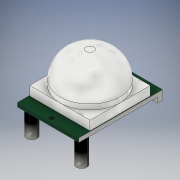
# Autodesk Inventor part: MotionSensor
Saved by Autodesk Inventor 2017.2 (Build 212223000, 223)
## iProperties
Created: 2017-02-21
Part Number: MotionSensor
Material: Generic
Document SubType Name: Modeling
Designer: prosp
Density: 1 g/cm^3
Appearance: Default
Author: prosp
Autodesk Inventor part; units mm, degrees
ref_plane "YZ Plane" through (0, 0, 0) normal (1, 0, 0) x (0, 1, 0)
ref_plane "XZ Plane" through (0, 0, 0) normal (0, 1, 0) x (-1, 0, 0)
ref_plane "XY Plane" through (0, 0, 0) normal (0, 0, 1) x (1, 0, 0)
sketch "Sketch1" plane through (0, 0, 0) normal (0, 1, 0) x (-1, 0, 0)
  line L0 (11.75, 16) -> (-11.75, 16)
  line L1 (-11.75, 16) -> (-11.75, -16)
  line L2 (-11.75, -16) -> (11.75, -16)
  line L3 (11.75, -16) -> (11.75, 16)
  point P0 (0, 0)
  dimension "d0" = 23.5
  dimension "d1" = 32
  constraints: 8 end point, 2 parallel, 1 horizontal, 1 perpendicular
  measures "d0" distance of L2.end L1.end
  measures "d1" distance of L2.end L0.start
extrude "Extrusion1" add sketch "Sketch1" along normal blind 1.5
sketch "Sketch2" plane through (0, 1.5, 0) normal (0, 1, 0) x (1, 0, 0)
  line L0 (-11.5, 11.5) -> (11.5, 11.5)
  line L1 (11.5, 11.5) -> (11.5, -11.5)
  line L2 (11.5, -11.5) -> (-11.5, -11.5)
  line L3 (-11.5, -11.5) -> (-11.5, 11.5)
  line L4 (-11.5, 11.5) -> (11.5, -11.5) construction
  line L5 (11.5, 11.5) -> (-11.5, -11.5) construction
  point P0 (0, 0)
  dimension "d4" = 23
  dimension "d5" = 23
  constraints: 12 end point, 2 midpoint, 2 parallel, 1 horizontal, 1 perpendicular
  measures "d4" distance of L0.start L0.end
  measures "d5" distance of L0.end L1.end
extrude "Extrusion2" add sketch "Sketch2" along normal blind 3.5
sketch "Sketch3" plane through (0, 5, 0) normal (0, 1, 0) x (1, 0, 0)
  circle A0 centre (0, 0) radius 11.5
  dimension "d8" = 23
  constraints: 1 centre point, 1 coincident
  measures "d8" diameter of A0
extrude "Extrusion3" add sketch "Sketch3" along normal blind 12
fillet "Fillet1" radius 10 1 edges at (-11.5, 17, 0)
sketch "Sketch4" plane through (0, 0, 0) normal (0, -1, 0) x (1, 0, 0)
  line L0 (11.75, -16) -> (-11.75, -16) projected
  line L1 (-11.75, -16) -> (-11.75, 16) projected
  circle A0 centre (-11.75, -16) radius 2
  line L2 (-11.75, 16) -> (11.75, 16) projected
  circle A1 centre (-11.75, 16) radius 2
  circle A2 centre (11.75, 16) radius 2
  line L3 (11.75, -16) -> (4.75, -16)
  line L4 (4.75, -16) -> (4.75, -14)
  line L5 (4.75, -14) -> (11.75, -14)
  line L6 (11.75, -14) -> (11.75, -16)
  line L7 (11.75, 16) -> (11.75, -16) projected
  line L8 (4.75, -15.5) -> (3.0316, -15.5)
  point P0 (0, 0)
  dimension "d13" = 4
  dimension "d14" = 4
  dimension "d20" = 4
  dimension "d21" = 7
  dimension "d22" = 2
  dimension "d36" = 0.5
  constraints: 10 end point, 3 centre point, 2 coincident, 1 point on line
  measures "d13" diameter of A0
  measures "d14" diameter of A1
  measures "d20" diameter of A2
  measures "d21" distance of L3.start L3.end
  measures "d22" distance of L3.end L4.end
  measures "d36" distance of L3.end L8.start
sketch "Sketch5" plane through (0, 0, 0) normal (0, -1, 0) x (1, 0, 0)
  line L0 (-9.743, 3.5) -> (-9.743, -3.5)
  line L1 (-9.743, -3.5) -> (-11.743, -3.5)
  line L2 (-11.743, -3.5) -> (-11.743, 3.5)
  line L3 (-11.743, 3.5) -> (-9.743, 3.5)
  line L4 (-11.75, -16) -> (-11.75, 16) projected
  point P0 (0, 0)
  point P1 (-11.75, 0)
  dimension "d16" = 7
  dimension "d17" = 2
  constraints: 8 end point, 2 parallel, 1 midpoint, 1 perpendicular
  measures "d16" distance of L0.start L0.end
  measures "d17" distance of L0.end L1.end
extrude "Extrusion4" add sketch "Sketch5" along normal blind 2
extrude "Extrusion5" add sketch "Sketch4" along normal blind 2 contours L0 L4 L5 L6
sketch "Sketch6" plane through (0, 0, 0) normal (0, -1, 0) x (1, 0, 0)
  circle A0 centre (9.525, 12.7) radius 2
  circle A1 centre (-9.525, 12.7) radius 2
  circle A2 centre (-9.525, -12.7) radius 2
  point P0 (0, 0)
  dimension "d26" = 4
  dimension "d27" = 4
  dimension "d28" = 4
  constraints: 3 centre point
  measures "d26" diameter of A0
  measures "d27" diameter of A1
  measures "d28" diameter of A2
extrude "Extrusion6" add sketch "Sketch6" along normal blind 10
sketch "Sketch7" plane through (0, -2, 0) normal (0, -1, 0) x (1, 0, 0)
  circle A0 centre (-10.8242, 0) radius 0.25
  circle A1 centre (-10.8242, 2.1954) radius 0.25
  circle A2 centre (-10.8242, -1.9618) radius 0.25
  point P0 (0, 0)
  dimension "d31" = 0.5
  dimension "d32" = 0.5
  dimension "d33" = 0.5
  constraints: 3 centre point
  measures "d31" diameter of A0
  measures "d32" diameter of A1
  measures "d33" diameter of A2
extrude "Extrusion7" add sketch "Sketch7" along normal blind 8
sketch "Sketch8" plane through (0, 1.5, 0) normal (0, 1, 0) x (1, 0, 0)
  circle A0 centre (0, 14.5) radius 1
  line L0 (0, 11.5) -> (-11.5, 11.5) projected
  circle A1 centre (0, -14.5) radius 1
  line L1 (-11.5, -11.5) -> (0, -11.5) projected
  point P0 (0, 0)
  dimension "d37" = 2
  dimension "d38" = 2
  constraints: 2 centre point
  measures "d37" diameter of A0
  measures "d38" diameter of A1
hole "Hole1" at (0, 1.5, -14.5) at (0, 1.5, 14.5) direction (0, -1, 0) diameter 2 end through all
body "Solid1"
